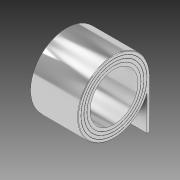
# Autodesk Inventor part: GreyT Constant Force Spring
Saved by Autodesk Inventor 2023 (Build 270158000, 158)
## iProperties
Created: 2022-01-24
Part Number: GreyT Constant Force Spring
Material: Steel
Document SubType Name: Modeling
Designer: Desktop
Density: 7.85 g/cm^3
Appearance: Chrome - Polished
Mass: 24.2764 g
Surface Area: 31.0148 cm^2
Volume: 3.09253 cm^3
Author: Desktop
Mass: 48.5361 g
Surface Area: 56.7995 cm^2
Volume: 6.18295 cm^3
Mass: 36.4149 g
Surface Area: 43.9937 cm^2
Volume: 4.63884 cm^3
Autodesk Inventor part; units mm, degrees
ref_plane "YZ Plane" through (0, 0, 0) normal (1, 0, 0) x (0, 1, 0)
ref_plane "XZ Plane" through (0, 0, 0) normal (0, 1, 0) x (-1, 0, 0)
ref_plane "XY Plane" through (0, 0, 0) normal (0, 0, 1) x (1, 0, 0)
sketch "Sketch1" plane through (0, 0, 0) normal (1, 0, 0) x (0, 1, 0)
  circle A0 centre (0, 0) radius 9.525
  circle A1 centre (0, 0) radius 8.7313
  line L0 (0, -9.525) -> (-12.7, -9.525)
  line L1 (-12.7, -9.525) -> (-12.7, -8.7313)
  line L2 (-12.7, -8.7313) -> (0, -8.7313)
  circle A2 centre (0, 0) radius 7.9375
  circle A3 centre (0, 0) radius 7.1438
  circle A4 centre (0, 0) radius 6.35
  point P0 (-3.8067, -8.7313)
  dimension "d13" = 19.05
  dimension "d0" = 0.7937
  dimension "d2" = 12.7
  dimension "d15" = 0.7937
  dimension "d16" = 0.7937
  dimension "d17" = 0.7937
  constraints: 6 end point, 4 horizontal, 3 centre point, 1 coincident, 1 perpendicular, 1 vertical alignment, 5 other
  measures "d0" distance between parallel lines of L0 L2
  measures "d2" distance of L0.start L0.end
  measures "d16" radial gap between concentric circles of A3 A2
  measures "d17" radial gap between concentric circles of A4 A3
extrude "Extrusion1" add sketch "Sketch1" along normal mid plane 12.7 contours A0 | L0 L1 L2 A0
chamfer "Chamfer2" distance 0.0254 angle 45 2 edges at (6.35, -8.7313, 0) (-6.35, -8.7313, 0)
extrude "Extrusion2" add sketch "Sketch1" along normal mid plane 12.7 contours A1
chamfer "Chamfer3" distance 0.0254 angle 45 4 edges at (-6.35, -8.7313, 0) (-6.35, -7.9375, 0) (6.35, -7.9375, 0) (6.35, -8.7313, 0)
extrude "Extrusion3" add sketch "Sketch1" along normal mid plane 12.7 contours A2
chamfer "Chamfer4" distance 0.0254 angle 45 4 edges at (-6.35, -7.9375, 0) (-6.35, -7.1438, 0) (6.35, -7.1438, 0) (6.35, -7.9375, 0)
extrude "Extrusion4" add sketch "Sketch1" along normal mid plane 12.7 contours A3
chamfer "Chamfer5" distance 0.0254 angle 45 1 edges at (-6.35, -7.1438, 0)
chamfer "Chamfer6" distance 0.127 angle 45 4 edges at (6.35, 1.9443, 9.3245) (6.35, -6.35, -9.525) (-6.35, 1.9443, 9.3245) (-6.35, -6.35, -9.525)
equation "\"d16\" = d15"
equation "\"d18\" = d3"
equation "\"d22\" = d8"
equation "\"d20\" = d3"
equation "\"d25\" = d8"
equation "\"d28\" = d3"
equation "\"d30\" = d8"
equation "\"d3\" = 12.7"
equation "\"d8\" = 0.0254"
body "Solid1"
